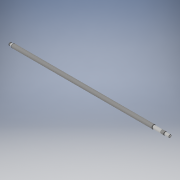
# Autodesk Inventor part: C-TBSE1204-500_t
Saved by Autodesk Inventor 2021 (Build 250183000, 183)
## iProperties
Created: 2023-01-12
Part Number: C-TBSE1204-500_t
Material: Generic
Catalog Web Link: www.cadenas.de
Description: C-TBSE1204, C-TBSE1205, C-TBSE1210, C-TBSB1204, C-TBSB1205, C-TBSB1210_thread-Economy Rolled Ball Screws - Thread Diameter 12, Lead 4/5/10 Precision Grade C7
Vendor: MISUMI
Document SubType Name: Modeling
Designer: psAdmin
Manufacturer: MISUMI
Mass: 53.714 g
Surface Area: 184.813 cm^2
Volume: 53.714 cm^3
Density: 1 g/cm^3
Appearance: PSOLRGB-175-175-175
Category: PARTsolutions
Company: MISUMI
PSOL_IDENT_0: {$CADENAS_DATA/23d-libs/misumi/metric/09_ball_screws/c_tbse12/c_tbse12_thread.prj},376 {VTYP=3D},{NB=
PSOL_IDENT_1: C-TBSE1204-500_t},{LINA=C-TBSE1204-500},{NN=C-TBSE1204, C-TBSE1205, C-TBSE1210, C-TBSB1204, C-TBSB12
PSOL_IDENT_2: 05, C-TBSB1210_thread},{DATE=21.09.2022 00:20:10},{GEOMDATE=19.11.2021 09:55:37},{VERSION=},{LINEID=
PSOL_IDENT_3: 30},{WBVAR=TS,LEAD,L,ALT3,ALT4,ALT2,ALT9,Q,G,ALT1,FC,ALT8,ALT10,ALT11,F1,P1,ALT5,KC,ALT6,K,S,ALT7,SC
PSOL_IDENT_4: ,ALT12,E1,U,ALT13},{WBNUMERIC=L,Q,G,FC,F1,P1,KC,K,S,SC,E1,U}  {NB=C-TBSE1204-500_t},{LINA=C-TBSE1204
PSOL_IDENT_5: -500},{KT=DUMMY},{PN=C-TBSE1204-500},{TS=E},{TYPE=C-TBSE},{AG=C7},{THRD=12},{LEAD=04},{L=500},{Y=439
PSOL_IDENT_6: },{A=35},{B=28.0},{T=8},{H=42},{C=32},{V=30},{LEAD1=4},{NUT=44.0},{ALT3=},{ALT33= '','w/o NC (No Mac
PSOL_IDENT_7: hining on Support Side Thread End)','-NC','with NC (No Machining on Support Side Thread End)'},{ALT4=
PSOL_IDENT_8: },{ALT4ALG= '', 'w/o RLC (Nut Direction)', '-RLC', 'with RLC (Nut Direction)' },{ALT2=},{ALT22= '','
PSOL_IDENT_9: w/o RNC (No Retaining Ring Groove on Support Side Thread End)','-RNC','with RNC (No Retaining Ring G
PSOL_IDENT_10: roove on Support Side Thread End)'},{ALT9=},{ALT9A='','w/o GC (Machining on Support Side Thread)','-
PSOL_IDENT_11: GC','with GC (Machining on Support Side Thread)'},{Q=0},{Q1=0},{Q2=},{G=0},{G1=0},{G2=0},{G3=},{ALT1=
PSOL_IDENT_12: },{ALT1ALG='','w/o FC (Support Side Thread End Length)','-FC','with FC (Support Side Thread End Leng
PSOL_IDENT_13: th)'},{FC=0},{FC1=[0:0/1]},{FC2=},{ALT8=},{ALT8ALG= '','w/o SZC (Fixed Side Wrench Flats Machining)'
PSOL_IDENT_14: , '-SZC'  , 'with SZC (Fixed Side Wrench Flats Machining)' },{ALT10=},{ALT10ALG= '','w/o NF (Fixed s
PSOL_IDENT_15: ide 1st stage No shaft end processing)','-NF','with NF (Fixed side 1st stage No shaft end processing
PSOL_IDENT_16: )'},{ALT11=},{ALT11ALG= '','w/o FP (Fixed side 1st step dimension change)','-FP','with FP (Fixed sid
PSOL_IDENT_17: e 1st step dimension change)'},{F=15},{F1=0},{FALG=0},{FMAX=24.000},{F2=},{P=8},{P1=0},{PALG=0},{P2=
PSOL_IDENT_18: },{ALT5=},{ALT5A= '', 'w/o KC (Key Groove on Fixed Side Thread End)', '-KC'  , 'with KC (Key Groove
PSOL_IDENT_19: on Fixed Side Thread End)' },{KC=0},{KC1=[0:0/1]},{KC2=},{KCMAX=14},{ALT6=},{ALT66= '','w/o KLC (Key
PSOL_IDENT_20: Groove on Fixed Side Thread End)','-KLC','with KLC (Key Groove on Fixed Side Thread End)'},{K=0},{K
PSOL_IDENT_21: 1=[0:0/1]},{K2=},{KMAX=13},{S=0},{SMAX=14},{S1=[0:0/1]},{S2=},{ALT7=},{ALT77= '', 'w/o SC (Fixed Par
PSOL_IDENT_22: t Thread End Flat Machining)', '-SC'  , 'with SC (Fixed Part Thread End Flat Machining)' },{SC=0},{S
PSOL_IDENT_23: C1=},{SC2=[0:0/1]},{SCMAX=14},{ALT12=},{ALT12ALG= '', 'w/o EU (Fixed side 2nd step Dimension change)'
PSOL_IDENT_24: , '-EU'  , 'with EU (Fixed side 2nd step Dimension change)' },{ALT12PN=},{E=36},{E1=0},{EALG=0},{EMI
PSOL_IDENT_25: N=11},{EMAX=40},{U=0},{U1=11},{UALG=0},{UMAX=33},{ALT13=},{ALT13ALG= '','w/o NU (No processing on th
PSOL_IDENT_26: e second set screw on the fixed side)','-NU','with NU (No processing on the second set screw on the
PSOL_IDENT_27: fixed side)'},{NDM=12.000},{KDM=10},{BB=3},{TT=1.2},{A1=7.6},{A2=8},{A3=0.9},{A4=7.9},{A5=10},{A6=24
PSOL_IDENT_28: },{C1=0.5},{R=0.3},{B1=10},{B2=26},{B3=11},{B4=10},{B5=12},{B6=8},{M=6},{PITCH=1.0},{NL=35},{LCOLLAR=
PSOL_IDENT_29: 449.0}
NB: C-TBSE1204-500_t
NN: C-TBSE1204, C-TBSE1205, C-TBSE1210, C-TBSB1204, C-TBSB1205, C-TBSB1210_thread
NT: Economy Rolled Ball Screws - Thread Diameter 12, Lead 4/5/10 Precision Grade C7
NBSYN: $PN._t
LINA: C-TBSE1204-500
CATALOG: Misumi
PN: C-TBSE1204-500
TS: EK Type
TYPE: C-TBSE
AG: C7
THRD: 12
LEAD: 04
L: 500
Y: 439
ALT3: w/o NC (No Machining on Support Side Thread End)
ALT4: w/o RLC (Nut Direction)
ALT2: w/o RNC (No Retaining Ring Groove on Support Side Thread End)
ALT9: w/o GC (Machining on Support Side Thread)
Q: 0
G: 0
ALT1: w/o FC (Support Side Thread End Length)
FC: 0
ALT8: w/o SZC (Fixed Side Wrench Flats Machining)
ALT10: w/o NF (Fixed side 1st stage No shaft end processing)
ALT11: w/o FP (Fixed side 1st step dimension change)
F1: 0
P1: 0
ALT5: w/o KC (Key Groove on Fixed Side Thread End)
KC: 0
ALT6: w/o KLC (Key Groove on Fixed Side Thread End)
K: 0
S: 0
ALT7: w/o SC (Fixed Part Thread End Flat Machining)
SC: 0
ALT12: w/o EU (Fixed side 2nd step Dimension change)
E1: 0
U: 0
ALT13: w/o NU (No processing on the second set screw on the fixed side)
SUPPLIER: MISUMI
ARTICLENO: C-TBSE1204-500_t
BOMINFO: C-TBSE1204-500
CREATOR: CADENAS GmbH
Title: C-TBSE1204-500
Author: Cadenas PARTsolutions
Comments: Economy Rolled Ball Screws - Thread Diameter 12, Lead 4/5/10 Precision Grade C7
Autodesk Inventor part; units mm, degrees
sketch "Sketch_1" plane through (0, 0, 0) normal (0, 0, 1) x (1, 0, 0)
  line L0 (449.5, 0) -> (0, 0)
  line L1 (0, 0) -> (0, 3.5)
  line L2 (0, 3.5) -> (0.5, 4)
  line L3 (0.5, 4) -> (2.1, 4)
  line L4 (2.1, 4) -> (2.1, 3.8)
  line L5 (2.1, 3.8) -> (3, 3.8)
  line L6 (3, 3.8) -> (3, 4)
  line L7 (3, 4) -> (9.5, 4)
  arc A0 (9.5, 4) -> (10, 4.5) centre (9.5, 4.5) ccw
  line L8 (10, 4.5) -> (10, 5.5)
  line L9 (10, 5.5) -> (10.5, 6)
  line L10 (10.5, 6) -> (448.5, 6)
  line L11 (448.5, 6) -> (449, 5.5)
  arc A1 (449, 5.5) -> (449.5, 5) centre (449.5, 5.5) ccw
  line L12 (449.5, 5) -> (449.5, 0)
  line L13 (449.5, 0) -> (0, 0)
  constraints: 28 end point, 4 point on circle, 2 centre point
revolve "Revolution1" add sketch "Sketch_1" angle 360 about axis through (449.5, 0, 0) along (1, 0, 0)
thread "Thread1" size "M12x1.5" class "6g" standard "ISO Metric profile" full length
sketch "_____2" plane through (0, 0, 0) normal (0, 0, 1) x (1, 0, 0)
  line L0 (500, 0) -> (449.5, 0)
  line L1 (449.5, 0) -> (449.5, 5)
  line L2 (449.5, 5) -> (484.5, 5)
  line L3 (484.5, 5) -> (485, 4.5)
  line L4 (485, 4.5) -> (485, 4.3)
  arc A0 (485, 4.3) -> (485.3, 4) centre (485.3, 4.3) ccw
  line L5 (485.3, 4) -> (499.5, 4)
  line L6 (499.5, 4) -> (500, 3.5)
  line L7 (500, 3.5) -> (500, 0)
  line L8 (500, 0) -> (449.5, 0)
  constraints: 18 end point, 2 point on circle, 1 centre point
revolve "Revolution2" add sketch "_____2" angle 360 about axis through (500, 0, 0) along (1, 0, 0)
thread "Thread2" size "M10x1" class "6g" standard "ISO Metric profile" length 10.5
ref_plane "to_collar_XY" through (449, 0, 0) normal (1, 0, 0) x (0, 0, -1)
ref_plane "to_collar_YZ" through (449, 0, 0) normal (0, 0, -1) x (0, 1, 0)
ref_plane "to_collar_ZX" through (449, 0, 0) normal (0, 1, 0) x (1, 0, 0)
ref_plane "to_dummy_XY" through (10, 0, 0) normal (1, 0, 0) x (0, 0, -1)
ref_plane "to_dummy_YZ" through (10, 0, 0) normal (0, 0, -1) x (0, 1, 0)
ref_plane "to_dummy_ZX" through (10, 0, 0) normal (0, 1, 0) x (1, 0, 0)
ref_plane "to_nut_XY" through (229.5, 0, 0) normal (1, 0, 0) x (0, 0, -1)
ref_plane "to_nut_YZ" through (229.5, 0, 0) normal (0, 0, -1) x (0, 1, 0)
ref_plane "to_nut_ZX" through (229.5, 0, 0) normal (0, 1, 0) x (1, 0, 0)
body "Solid1"
